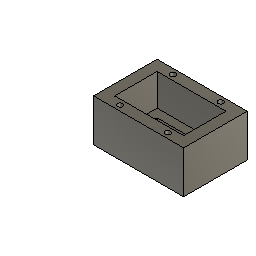
Base (Autodesk Fusion 360 design; units mm, degrees)
Autodesk Fusion 360 part; units mm, degrees
sketch "Sketch3" plane through (0, 0, 0) normal (0, 0, 1) x (1, 0, 0)
  line L0 (-10, 50) -> (75, 50)
  line L1 (75, 50) -> (75, 40)
  line L2 (65, 40) -> (0, 40)
  line L3 (-10, 40) -> (-10, 50)
  line L4 (75, -10) -> (65, -10)
  line L5 (65, 0) -> (65, 40)
  line L6 (75, 40) -> (75, -10)
  line L7 (65, -10) -> (-10, -10)
  line L8 (-10, -10) -> (-10, 0)
  line L9 (0, 0) -> (65, 0)
  line L10 (0, 0) -> (0, 40)
  line L11 (-10, 40) -> (-10, 0)
  constraint horizontal L0
  constraint vertical L1
  constraint horizontal L2
  constraint vertical L3
  constraint horizontal L4
  constraint vertical L5
  constraint vertical L6
  constraint horizontal L7
  constraint vertical L8
  constraint horizontal L9
  constraint vertical L10
  constraint vertical L11
sketch "Sketch1" plane through (0, 0, 0) normal (0, 0, 1) x (1, 0, 0)
  line L0 (0, 0) -> (65, 0)
  line L1 (65, 0) -> (65, 40)
  line L2 (65, 40) -> (0, 40)
  line L3 (0, 40) -> (0, 0)
  line L4 (8, 8) -> (57, 8)
  line L5 (57, 8) -> (57, 32)
  line L6 (57, 32) -> (8, 32)
  line L7 (8, 32) -> (8, 8)
  dimension "d1" = 65
  dimension "d2" = 40
  dimension "d3" = -8
  constraint horizontal L0
  constraint vertical L1
  constraint horizontal L2
  constraint vertical L3
  constraint coincident L0.start L3.end
  measures "d1" distance of L0.start L0.end
  measures "d2" distance of L0.start L2.end
extrude "Extrude1" add sketch "Sketch1" along normal blind 10 makes body 1
extrude "Extrude2" add sketch "Sketch3" along normal blind 40 bodies 1
copy_body "CutPasteBodies1" bodies 1 removing the originals makes body 2
sketch "Sketch1 (1)" plane through (0, 0, 40) normal (0, 0, 1) x (-1, 0, 0)
  line L0 (-65, -40) -> (-65, 0)
  line L1 (-65, 0) -> (0, 0)
  line L2 (0, 0) -> (0, -40)
  line L3 (0, -40) -> (-65, -40)
  line L4 (10, -50) -> (10, 10)
  line L5 (10, 10) -> (-75, 10)
  line L6 (-75, 10) -> (-75, -50)
  line L7 (-75, -50) -> (10, -50)
  circle A0 centre (-55, -45) radius 2.5
  circle A1 centre (-10, -45) radius 2.5
  circle A2 centre (-10, 5) radius 2.5
  circle A3 centre (-55, 5) radius 2.5
  dimension "d17" = 5
  dimension "d18" = 5
  dimension "d19" = 5
  dimension "d20" = 5
  measures "d17" diameter of A0
  measures "d18" diameter of A1
  measures "d19" diameter of A2
  measures "d20" diameter of A3
extrude "Extrude1'" cut sketch "Sketch1 (1)" against normal blind 10 contours A0 | A1 | A2 | A3 bodies 2
